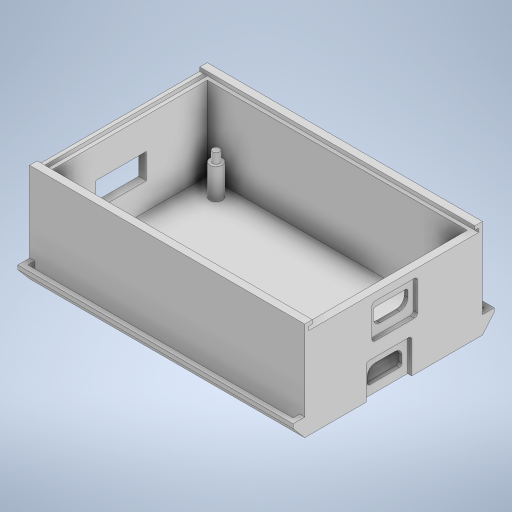
# Autodesk Inventor part: ControllerChassis
Saved by Autodesk Inventor 2024 (Build 280153000, 153)
## iProperties
Created: 2024-03-27
Part Number: ControllerChassis
Material: Generic
Document SubType Name: Modeling
Designer: bbbmi
Density: 1 g/cm^3
Appearance: Default
Author: bbbmi
Autodesk Inventor part; units mm, degrees
ref_plane "YZ Plane" through (0, 0, 0) normal (1, 0, 0) x (0, 1, 0)
ref_plane "XZ Plane" through (0, 0, 0) normal (0, 1, 0) x (-1, 0, 0)
ref_plane "XY Plane" through (0, 0, 0) normal (0, 0, 1) x (1, 0, 0)
sketch "Sketch1" plane through (0, 0, 0) normal (0, 1, 0) x (-1, 0, 0)
  circle A0 centre (57.0611, -2.9464) radius 0.889
  circle A1 centre (57.0611, -36.957) radius 0.889
  circle A2 centre (2.9464, -2.9464) radius 0.889
  circle A3 centre (2.9464, -36.957) radius 0.889
  line L0 (0, -39.9034) -> (-2.0828, -39.9034)
  line L1 (-2.0828, 0) -> (-2.0828, -39.9034)
  line L2 (-2.0828, 0) -> (-2.0828, -39.9034)
  line L3 (-2.0828, -39.9034) -> (62.2173, -39.9034)
  line L4 (62.2173, -39.9034) -> (62.2173, 0)
  line L5 (-2.0828, 0) -> (62.2173, 0)
  line L6 (62.6142, 0.3969) -> (62.6142, -40.3003)
  line L7 (62.6142, -40.3003) -> (-2.4797, -40.3003)
  line L8 (-2.4797, -40.3003) -> (-2.4797, 0.3969)
  line L9 (-2.4797, 0.3969) -> (62.6142, 0.3969)
  circle A4 centre (2.9464, -2.9464) radius 1.5875
  circle A5 centre (2.9464, -36.957) radius 1.5875
  circle A6 centre (57.0611, -36.957) radius 1.5875
  circle A7 centre (57.0611, -2.9464) radius 1.5875
  line L10 (64.5192, -42.2053) -> (64.5192, 2.3019)
  line L11 (64.5192, 2.3019) -> (-4.3847, 2.3019)
  line L12 (-4.3847, 2.3019) -> (-4.3847, -42.2053)
  line L13 (-4.3847, -42.2053) -> (64.5192, -42.2053)
  point P0 (0, 0)
  dimension "d3" = 1.778
  dimension "d4" = 1.778
  dimension "d5" = 1.778
  dimension "d6" = 1.778
  dimension "d7" = 2.0828
  dimension "d9" = 0.3969
  dimension "d10" = 3.175
  dimension "d11" = 3.175
  dimension "d12" = 3.175
  dimension "d13" = 3.175
  dimension "d14" = 65.0939
  dimension "d15" = 1.905
  constraints: 28 end point, 8 centre point, 4 coincident, 3 parallel, 3 perpendicular, 6 other
  measures "d3" diameter of A0
  measures "d4" diameter of A1
  measures "d5" diameter of A2
  measures "d6" diameter of A3
  measures "d7" distance of L0.start L0.end
  measures "d9" distance between parallel lines of L5 L9
  measures "d10" diameter of A4
  measures "d11" diameter of A5
  measures "d12" diameter of A6
  measures "d13" diameter of A7
  measures "d14" distance of L8.end L6.start
  measures "d15" distance between parallel lines of L6 L10
extrude "Extrusion1" add sketch "Sketch1" against normal blind 1.905 contours A0 | A1 | A2 | A3 | L0 L1 L5 L4 L3 | L6 L7 L8 L9 | A4 | A5 | A6 | A7 | L13 L12 L11 L10
extrude "Extrusion2" add sketch "Sketch1" along normal blind 20.32 contours L13 L12 L11 L10
extrude "Extrusion3" add sketch "Sketch1" along normal blind 7.62 contours A0 | A1 | A2 | A3 | A4 | A5 | A6 | A7
extrude "Extrusion4" add sketch "Sketch1" along normal blind 10.16 contours A0 | A1 | A2 | A3
sketch "Sketch2" plane through (-62.6142, 0, -40.3003) normal (1, 0, 0) x (0, 0, -1)
  line L0 (-35.7664, 7.62) -> (-38.9414, 7.62) projected
  line L1 (-1.7558, 7.62) -> (-4.9308, 7.62) projected
  line L2 (-38.9414, 7.62) -> (-1.7558, 7.62) construction
  line L3 (-0.1345, 12.2585) -> (-15.2729, 12.2585) construction
  line L4 (-40.6972, 0) -> (-40.6972, 20.32) construction
  line L5 (-40.6972, 12.2585) -> (-27.9972, 12.2585) construction
  line L6 (-40.6972, 12.2585) -> (-27.9972, 12.2585) construction
  line L7 (-29.9766, 7.62) -> (-29.9766, 12.827) construction
  line L8 (-12.5123, 13.2239) -> (-30.3735, 13.2239) construction
  line L9 (-30.3735, 13.2239) -> (-30.3735, 7.62) construction
  line L10 (-27.9972, 15.5048) -> (-27.9972, 4.9416) construction
  line L11 (-15.2729, 15.5048) -> (-15.2729, 4.9416) construction
  line L12 (-26.1455, 7.62) -> (-26.1455, 6.858) construction
  line L13 (-26.1455, 6.858) -> (-26.1455, 6.4611) construction
  line L14 (-26.1455, 6.4611) -> (-27.9972, 6.4611) construction
  line L15 (-27.9972, 6.4611) -> (-15.2729, 6.4611) construction
  line L16 (-27.9972, 13.2239) -> (-15.2729, 13.2239)
  line L17 (-15.2729, 13.2239) -> (-15.2729, 6.4611)
  line L18 (-15.2729, 6.4611) -> (-27.9972, 6.4611)
  line L19 (-27.9972, 6.4611) -> (-27.9972, 13.2239)
  point P0 (-40.3003, 0)
  dimension "d24" = 15.1384
  dimension "d25" = 12.7
  dimension "d26" = 0
  dimension "d27" = 12.7242
  dimension "d28" = 5.207
  dimension "d30" = 0.762
  dimension "d31" = 0.3969
  constraints: 34 end point, 9 point on line, 6 perpendicular, 3 horizontal, 2 collinear, 2 parallel
  measures "d24" distance of L3.start L3.end
  measures "d25" distance of L5.start L5.end
  measures "d26" distance between parallel lines of L5 L6
  measures "d27" distance of L3.end L5.end
  measures "d28" distance of L7.start L7.end
  measures "d30" distance of L12.start L12.end
  measures "d31" distance of L12.end L13.end
extrude "Extrusion5" cut sketch "Sketch2" against normal blind 10.16
sketch "Sketch3" plane through (-62.6142, 6.4611, -12.3031) normal (0, 1, 0) x (1, 0, 0)
  line L0 (-1.905, 0) -> (-1.905, 12.7242) projected
  line L1 (0, 0) -> (-1.905, 0) projected
  line L2 (0, 12.7242) -> (0, 0) projected
  line L3 (0, 12.7242) -> (-1.905, 12.7242) projected
  point P0 (62.6142, -12.3031)
extrude "Extrusion6" add sketch "Sketch3" along normal blind 0.2032
sketch "Sketch4" plane through (-62.6142, 13.2239, -25.0273) normal (0, -1, 0) x (1, 0, 0)
  line L0 (-1.905, 0) -> (-1.905, 12.7242) projected
  line L1 (0, 0) -> (-1.905, 0) projected
  line L2 (0, 12.7242) -> (0, 0) projected
  line L3 (0, 12.7242) -> (-1.905, 12.7242) projected
  point P0 (62.6142, 25.0273)
extrude "Extrusion7" add sketch "Sketch4" along normal blind 0.2032
sketch "Sketch5" plane through (2.4797, 0, 0.3969) normal (-1, 0, 0) x (0, 0, 1)
  line L0 (-35.7664, 7.62) -> (-38.9414, 7.62) projected
  line L1 (-1.7558, 7.62) -> (-4.9308, 7.62) projected
  line L2 (0, 0) -> (0, 20.32) projected
  line L3 (0, 0) -> (-40.6972, 0) projected
  line L4 (0, 0) -> (0, 20.32) projected
  line L5 (-40.6972, 20.32) -> (0, 20.32) projected
  line L6 (-40.6972, 0) -> (-40.6972, 20.32) projected
  line L7 (0, 17.9413) -> (-16.256, 17.9413) construction
  line L8 (-40.6972, 17.9413) -> (-24.9492, 17.9413) construction
  line L9 (-38.9414, 7.62) -> (-1.7558, 7.62) construction
  line L10 (-31.4008, 7.62) -> (-31.4008, 16.637) construction
  line L11 (-31.4008, 16.637) -> (-9.7411, 16.637) construction
  line L12 (-11.2605, 7.62) -> (-11.2605, 12.5984) construction
  line L13 (-11.2605, 12.5984) -> (-27.4568, 12.5984) construction
  line L14 (-24.9492, 16.002) -> (-24.9492, 11.6374) construction
  line L15 (-16.256, 17.9413) -> (-16.256, 10.1092) construction
  line L16 (-24.3142, 16.637) -> (-16.891, 16.637)
  line L17 (-16.256, 16.002) -> (-16.256, 12.5984)
  line L18 (-16.256, 12.5984) -> (-24.9492, 12.5984)
  line L19 (-24.9492, 12.5984) -> (-24.9492, 16.637)
  arc A0 (-24.9492, 14.6177) -> (-22.9299, 12.5984) centre (-22.9299, 14.6177) ccw
  line L20 (-24.9492, 14.6177) -> (-22.9299, 12.5984) construction
  line L21 (-24.9492, 14.6177) -> (-22.0934, 14.6177) construction
  arc A1 (-17.9578, 12.5984) -> (-16.256, 14.3002) centre (-17.9578, 14.3002) ccw
  line L22 (-16.256, 14.3002) -> (-17.9578, 12.5984) construction
  line L23 (-16.256, 14.3002) -> (-13.8493, 14.3002) construction
  arc A2 (-24.3142, 16.637) -> (-24.9492, 16.002) centre (-24.3142, 16.002) ccw
  arc A3 (-16.256, 16.002) -> (-16.891, 16.637) centre (-16.891, 16.002) ccw
  line L24 (-15.367, 0.4545) -> (-22.7902, 0.4545)
  line L25 (-23.4252, 1.0895) -> (-23.4252, 4.4931)
  line L26 (-23.4252, 4.4931) -> (-14.732, 4.4931)
  line L27 (-14.732, 4.4931) -> (-14.732, 0.4545)
  arc A4 (-14.732, 2.4738) -> (-16.7513, 4.4931) centre (-16.7513, 2.4738) ccw
  line L28 (-14.732, 2.4738) -> (-16.7513, 4.4931) construction
  line L29 (-14.732, 2.4738) -> (-17.5877, 2.4738) construction
  arc A5 (-21.7234, 4.4931) -> (-23.4252, 2.7913) centre (-21.7234, 2.7913) ccw
  line L30 (-23.4252, 2.7913) -> (-21.7234, 4.4931) construction
  arc A6 (-15.367, 0.4545) -> (-14.732, 1.0895) centre (-15.367, 1.0895) ccw
  arc A7 (-23.4252, 1.0895) -> (-22.7902, 0.4545) centre (-22.7902, 1.0895) ccw
  line L31 (-35.7664, 7.62) -> (-35.7664, 3.9878) construction
  line L32 (-40.6972, 3.9878) -> (-23.222, 3.9878) construction
  line L33 (0, 1.7909) -> (-16.3322, 1.7909) construction
  line L34 (-28.4303, 7.62) -> (-28.4303, 0.8509) construction
  line L35 (-28.4303, 0.8509) -> (-22.4064, 0.8509) construction
  line L36 (0, 4.4931) -> (-14.732, 4.4931)
  point P0 (-0.3969, 0)
  point P1 (-14.732, 1.0895)
  dimension "d38" = 16.256
  dimension "d39" = 15.748
  dimension "d40" = 9.017
  dimension "d41" = 4.9784
  dimension "d42" = 45
  dimension "d43" = 135
  dimension "d44" = 0.635
  dimension "d45" = 45
  dimension "d46" = 0.635
  dimension "d47" = 3.6322
  dimension "d48" = 17.4752
  dimension "d49" = 16.3322
  dimension "d50" = 6.7691
  dimension "d157" = 14.732
  constraints: 60 end point, 19 point on line, 16 point on circle, 11 tangent, 10 perpendicular, 8 centre point, 5 horizontal, 4 midpoint, 4 parallel, 4 vertical, 3 equal length, 2 equal radius, 1 collinear
  measures "d38" distance of L7.start L7.end
  measures "d39" distance of L8.start L8.end
  measures "d40" distance of L10.start L10.end
  measures "d41" distance of L12.start L12.end
  measures "d42" angle of L20 L21
  measures "d43" angle of L22 L23
  measures "d44" radius of A2
  measures "d45" angle of L28 L29
  measures "d46" radius of A6
  measures "d47" distance of L0.start L31.end
  measures "d48" distance of L32.start L32.end
  measures "d49" distance of L33.start L33.end
  measures "d50" distance of L34.start L34.end
  measures "d157" distance of L36.start L36.end
extrude "Extrusion8" cut sketch "Sketch5" against normal blind 25.4 contours L16 A3 L17 A1 L18 A0 L19 A2 | L24 A7 L25 A5 L26 A4 L27 A6
sketch "Sketch6" plane through (0, 20.32, 0) normal (0, 1, 0) x (1, 0, 0)
  line L0 (-64.5192, -2.3019) -> (4.3847, -2.3019) projected
  line L1 (4.3847, -2.3019) -> (4.3847, 42.2053) projected
  line L2 (4.3847, 42.2053) -> (-64.5192, 42.2053) projected
  line L3 (-64.5192, 42.2053) -> (-64.5192, -2.3019) projected
  line L4 (-62.6142, -0.3969) -> (-62.6142, 40.3003) projected
  line L5 (-62.6142, 40.3003) -> (2.4797, 40.3003) projected
  line L6 (2.4797, 40.3003) -> (2.4797, -0.3969) projected
  line L7 (2.4797, -0.3969) -> (-62.6142, -0.3969) projected
  point P0 (0, 0)
extrude "Extrusion9" add sketch "Sketch6" along normal blind 0.508
sketch "Sketch7" plane through (0, 20.828, 0) normal (0, 1, 0) x (1, 0, 0)
  line L0 (4.3847, -2.3019) -> (4.3847, 42.2053) projected
  line L1 (4.3847, 42.2053) -> (-64.5192, 42.2053) projected
  line L2 (-64.5192, 42.2053) -> (-64.5192, -2.3019) projected
  line L3 (-64.5192, -2.3019) -> (4.3847, -2.3019) projected
  line L4 (-62.6142, -0.3969) -> (-62.6142, 40.3003) projected
  line L5 (-62.6142, 40.3003) -> (2.4797, 40.3003) projected
  line L6 (2.4797, 40.3003) -> (2.4797, -0.3969) projected
  line L7 (2.4797, -0.3969) -> (-62.6142, -0.3969) projected
  line L8 (-63.5667, -1.3494) -> (-63.5667, 41.2528)
  line L9 (-63.5667, 41.2528) -> (3.4322, 41.2528)
  line L10 (3.4322, 41.2528) -> (3.4322, -1.3494)
  line L11 (3.4322, -1.3494) -> (-63.5667, -1.3494)
  line L12 (3.4322, -1.3494) -> (4.3847, -1.3494)
  line L13 (3.4322, 41.2528) -> (4.3847, 41.2528)
  point P0 (0, 0)
  dimension "d55" = 0.9525
  constraints: 12 end point, 3 point on line, 1 perpendicular, 3 other
  measures "d55" distance between parallel lines of L7 L11
extrude "Extrusion10" add sketch "Sketch7" along normal blind 0.9525 contours L3 L2 L1 L0 L13 L9 L8 L11 L12
sketch "Sketch8" plane through (0, 21.7805, 0) normal (0, 1, 0) x (1, 0, 0)
  line L0 (4.3847, -1.3494) -> (-63.5667, -1.3494) projected
  line L1 (2.4688, -1.3494) -> (0.6908, -1.3494)
  arc A0 (0.6908, -1.3494) -> (2.4688, -1.3494) centre (1.5798, -1.3494) ccw
  line L2 (4.3847, 41.2528) -> (-63.5667, 41.2528) projected
  line L3 (2.4688, 41.2528) -> (0.6908, 41.2528)
  arc A1 (2.4688, 41.2528) -> (0.6908, 41.2528) centre (1.5798, 41.2528) ccw
  point P0 (0, 0)
  dimension "d58" = 1.778
  dimension "d59" = 0.889
  dimension "d60" = 1.778
  dimension "d61" = 0.889
  constraints: 4 end point, 4 point on circle, 4 point on line, 2 centre point
  measures "d58" distance of L1.start L1.end
  measures "d59" radius of A0
  measures "d60" distance of L3.start L3.end
  measures "d61" radius of A1
extrude "Extrusion11" cut sketch "Sketch8" against normal blind 0.9525
sketch "Sketch9" plane through (0, 21.7805, 0) normal (0, 1, 0) x (1, 0, 0)
  line L0 (-62.6142, -0.3969) -> (-62.6142, 40.3003) projected
  line L1 (-62.6142, 40.3003) -> (2.4797, 40.3003) projected
  line L2 (2.4797, 40.3003) -> (2.4797, -0.3969) projected
  line L3 (2.4797, -0.3969) -> (-62.6142, -0.3969) projected
  line L4 (4.3847, 41.2528) -> (2.4688, 41.2528) projected
  arc A0 (2.4688, 41.2528) -> (0.6908, 41.2528) centre (1.5798, 41.2528) ccw projected
  line L5 (0.6908, 41.2528) -> (-63.5667, 41.2528) projected
  line L6 (-63.5667, 41.2528) -> (-63.5667, -1.3494) projected
  line L7 (-63.5667, -1.3494) -> (0.6908, -1.3494) projected
  arc A1 (0.6908, -1.3494) -> (2.4688, -1.3494) centre (1.5798, -1.3494) ccw projected
  line L8 (2.4688, -1.3494) -> (4.3847, -1.3494) projected
  line L9 (4.3847, -1.3494) -> (4.3847, 41.2528) projected
  arc A2 (0.6908, -1.3494) -> (2.4688, -1.3494) centre (1.5798, -1.3494) ccw projected
  line L10 (0.6908, -1.3494) -> (-63.5667, -1.3494) projected
  line L11 (-63.5667, -1.3494) -> (-63.5667, 41.2528) projected
  line L12 (-63.5667, 41.2528) -> (0.6908, 41.2528) projected
  arc A3 (2.4688, 41.2528) -> (0.6908, 41.2528) centre (1.5798, 41.2528) ccw projected
  line L13 (2.4688, 41.2528) -> (4.3847, 41.2528) projected
  line L14 (4.3847, 41.2528) -> (4.3847, 42.2053) projected
  line L15 (4.3847, 42.2053) -> (-64.5192, 42.2053) projected
  line L16 (-64.5192, 42.2053) -> (-64.5192, -2.3019) projected
  line L17 (-64.5192, -2.3019) -> (4.3847, -2.3019) projected
  line L18 (4.3847, -2.3019) -> (4.3847, -1.3494) projected
  line L19 (4.3847, -1.3494) -> (2.4688, -1.3494) projected
  line L20 (2.4797, -0.3969) -> (4.3847, -0.3969)
  line L21 (2.4797, 40.3003) -> (-62.6142, 40.3003) projected
  line L22 (2.4797, 40.3003) -> (4.3847, 40.3003)
  line L23 (-63.5667, 41.2528) -> (-64.5192, 41.2528)
  line L24 (-64.5192, 42.2053) -> (-64.5192, -2.3019) projected
  line L25 (0.6908, -1.3494) -> (-63.5667, -1.3494) projected
  line L26 (-63.5667, -1.3494) -> (-64.5497, -1.3494)
  line L27 (-62.6142, 40.3003) -> (-64.5192, 40.3003)
  line L28 (-62.6142, 40.3003) -> (-60.7092, 40.3003) construction
  line L29 (-62.6142, -0.3969) -> (-62.6142, 40.3003) projected
  line L30 (-62.6142, -0.3969) -> (-64.5192, -0.3969)
  line L31 (-62.6142, -0.3969) -> (-60.7092, -0.3969) construction
  point P0 (0, 0)
  dimension "d64" = 180
  dimension "d65" = 180
  constraints: 16 end point, 5 point on line, 3 perpendicular, 2 collinear, 2 horizontal, 1 parallel
  measures "d64" angle of L27 L28
  measures "d65" angle of L30 L31
extrude "Extrusion12" add sketch "Sketch9" along normal blind 0.9525 contours L3 L20 L9 L8 A1 L7 L6 L30 | L27 L6 L5 A0 L4 L9 L22 L1 | L6 L26 L16 L30 | L27 L16 L23 L6 | L7 A1 L8 L18 L17 L16 L26 | L23 L16 L15 L14 L4 A0 L5
sketch "Sketch10" plane through (4.3847, -1.905, 2.3019) normal (1, 0, 0) x (0, 0, -1)
  line L0 (0, 0) -> (0, 24.638) projected
  line L1 (0, 0) -> (0, 4.4819)
  line L2 (-2.921, 4.4819) -> (-2.921, 3.4361)
  line L3 (-2.921, 3.4361) -> (0, 0)
  line L4 (-2.921, 4.4819) -> (-1.651, 4.4819)
  line L5 (-1.1001, 3.255) -> (0, 1.9608)
  line L6 (-1.1001, 3.255) -> (-1.651, 3.903)
  line L7 (-1.651, 3.903) -> (-1.651, 4.4819)
  line L8 (-1.651, 3.903) -> (0, 1.9608)
  line L9 (-1.651, 4.4819) -> (-2.921, 4.4819)
  line L10 (44.5071, 0) -> (44.5071, 4.4819)
  line L11 (47.4281, 4.4819) -> (47.4281, 3.4361)
  line L12 (47.4281, 3.4361) -> (44.5071, 0)
  line L13 (47.4281, 4.4819) -> (46.1581, 4.4819)
  line L14 (45.6073, 3.255) -> (44.5071, 1.9608)
  line L15 (45.6073, 3.255) -> (46.1581, 3.903)
  line L16 (46.1581, 3.903) -> (46.1581, 4.4819)
  line L17 (46.1581, 3.903) -> (44.5071, 1.9608)
  line L18 (46.1581, 4.4819) -> (47.4281, 4.4819)
  point P0 (2.3019, 1.905)
  point P1 (0, 1.9608)
  dimension "d69" = 2.921
  dimension "d70" = 1.27
  constraints: 36 end point, 5 point on line, 2 perpendicular, 1 collinear
  measures "d69" distance of L1.end L2.start
  measures "d70" distance of L2.start L4.end
extrude "Extrusion13" add sketch "Sketch10" against normal up to surface (68.9039 mm away)
sketch "Sketch11" plane through (4.3847, 20.828, 1.3494) normal (1, 0, 0) x (0, 0, -1)
  line L0 (-2.6035, -18.83) -> (-2.6035, -18.2511) projected
  line L1 (-0.9525, -20.7722) -> (-2.6035, -18.83) projected
  line L2 (-0.9525, -20.7722) -> (-0.9525, 1.905) projected
  line L3 (45.2056, -18.2511) -> (45.2056, -18.83) projected
  line L4 (45.2056, -18.83) -> (43.5546, -20.7722) projected
  line L5 (43.5546, -20.7722) -> (43.5546, 1.905) projected
  line L6 (45.2056, -18.2511) -> (43.5546, -18.2511)
  line L7 (-2.6035, -18.2511) -> (-3.8735, -18.2511) projected
  line L8 (-2.6035, -18.2511) -> (-0.9525, -18.2511)
  point P0 (1.3494, -20.828)
  constraints: 4 end point, 2 perpendicular, 2 point on line
extrude "Extrusion14" add sketch "Sketch11" against normal blind 1.27
sketch "Sketch12" plane through (-64.5192, 21.7805, -40.3003) normal (-1, 0, 0) x (0, 0, 1)
  line L0 (44.2531, -19.7825) -> (42.6021, -21.7247) projected
  line L1 (44.2531, -19.2036) -> (44.2531, -19.7825) projected
  line L2 (44.2531, -19.2036) -> (42.6021, -19.2036) projected
  line L3 (42.6021, -21.7247) -> (42.6021, -19.2036) projected
  line L4 (-3.556, -19.7825) -> (-3.556, -19.2036) projected
  line L5 (-1.905, -21.7247) -> (-3.556, -19.7825) projected
  line L6 (-1.905, -19.2036) -> (-1.905, -21.7247) projected
  line L7 (-1.905, -19.2036) -> (-3.556, -19.2036) projected
  point P0 (40.3003, -21.7805)
extrude "Extrusion15" add sketch "Sketch12" against normal blind 1.27
sketch "Sketch13" plane through (0, -1.905, 0) normal (0, -1, 0) x (1, 0, 0)
  line L0 (4.3847, 2.3019) -> (-64.5192, 2.3019) projected
  line L1 (-64.5192, 2.3019) -> (-64.5192, -42.2053) projected
  line L2 (-64.5192, -42.2053) -> (4.3847, -42.2053) projected
  line L3 (4.3847, -42.2053) -> (4.3847, 2.3019) projected
  circle A0 centre (-30.0673, -19.9517) radius 3.81
  circle A1 centre (-17.3673, -19.9517) radius 3.81
  circle A2 centre (-4.6673, -19.9517) radius 3.81
  circle A3 centre (-30.0673, -32.6517) radius 3.81
  circle A4 centre (-17.3673, -32.6517) radius 3.81
  circle A5 centre (-4.6673, -32.6517) radius 3.81
  circle A6 centre (-17.3673, -32.6517) radius 3.81
  circle A7 centre (-30.0673, -32.6517) radius 3.81
  circle A8 centre (-42.7673, -32.6517) radius 3.81
  circle A9 centre (-55.4673, -32.6517) radius 3.81
  circle A10 centre (-4.6673, -19.9517) radius 3.81
  circle A11 centre (-17.3673, -19.9517) radius 3.81
  circle A12 centre (-30.0673, -19.9517) radius 3.81
  circle A13 centre (-42.7673, -19.9517) radius 3.81
  circle A14 centre (-55.4673, -19.9517) radius 3.81
  circle A15 centre (-4.6673, -7.2517) radius 3.81
  circle A16 centre (-17.3673, -7.2517) radius 3.81
  circle A17 centre (-30.0673, -7.2517) radius 3.81
  circle A18 centre (-42.7673, -7.2517) radius 3.81
  circle A19 centre (-55.4673, -7.2517) radius 3.81
  point P0 (0, 0)
  dimension "d83" = 12.7
  dimension "d86" = 12.7
  dimension "d91" = 12.7
  dimension "d94" = 12.7
  constraints: 20 centre point, 2 horizontal, 2 vertical, 38 other
  measures "d83" distance of A0.centre A1.centre
  measures "d86" distance of A0.centre A3.centre
  measures "d91" distance of A5.centre A6.centre
  measures "d94" distance of A5.centre A10.centre
extrude "Extrusion16" add sketch "Sketch13" along normal blind 2.54 contours A0 | A1 | A2 | A3 | A4 | A5 | A8 | A9 | A13 | A14 | A15 | A16 | A17 | A18 | A19
chamfer "Chamfer1" distance 3.556 distance2 2.54 1 edges at (-8.4773, -4.445, -19.9517) measured on face at (-7.9773, -4.445, -19.9517)
chamfer "Chamfer2" distance 3.556 distance2 2.54 1 edges at (-8.4773, -4.445, -32.6517) measured on face at (-7.9773, -4.445, -32.6517)
chamfer "Chamfer3" distance 3.556 distance2 2.54 1 edges at (-21.1773, -4.445, -32.6517) measured on face at (-20.6773, -4.445, -32.6517)
chamfer "Chamfer4" distance 3.556 distance2 2.54 1 edges at (-33.8773, -4.445, -32.6517) measured on face at (-33.3773, -4.445, -32.6517)
chamfer "Chamfer5" distance 3.556 distance2 2.54 1 edges at (-46.5773, -4.445, -32.6517) measured on face at (-46.0773, -4.445, -32.6517)
chamfer "Chamfer6" distance 3.556 distance2 2.54 1 edges at (-59.2773, -4.445, -32.6517) measured on face at (-58.7773, -4.445, -32.6517)
chamfer "Chamfer7" distance 3.556 distance2 2.54 1 edges at (-21.1773, -4.445, -19.9517) measured on face at (-20.6773, -4.445, -19.9517)
chamfer "Chamfer8" distance 3.556 distance2 2.54 1 edges at (-33.8773, -4.445, -19.9517) measured on face at (-33.3773, -4.445, -19.9517)
chamfer "Chamfer9" distance 3.556 distance2 2.54 1 edges at (-46.5773, -4.445, -19.9517) measured on face at (-46.0773, -4.445, -19.9517)
chamfer "Chamfer10" distance 3.556 distance2 2.54 1 edges at (-8.4773, -4.445, -7.2517) measured on face at (-7.9773, -4.445, -7.2517)
chamfer "Chamfer11" distance 3.556 distance2 2.54 1 edges at (-21.1773, -4.445, -7.2517) measured on face at (-20.6773, -4.445, -7.2517)
chamfer "Chamfer12" distance 3.556 distance2 2.54 1 edges at (-33.8773, -4.445, -7.2517) measured on face at (-33.3773, -4.445, -7.2517)
chamfer "Chamfer13" distance 3.556 distance2 2.54 1 edges at (-59.2773, -4.445, -19.9517) measured on face at (-58.7773, -4.445, -19.9517)
chamfer "Chamfer14" distance 3.556 distance2 2.54 1 edges at (-46.5773, -4.445, -7.2517) measured on face at (-46.0773, -4.445, -7.2517)
chamfer "Chamfer15" distance 3.556 distance2 2.54 1 edges at (-59.2773, -4.445, -7.2517) measured on face at (-58.7773, -4.445, -7.2517)
sketch "Sketch14" plane through (0, -1.905, 0) normal (0, -1, 0) x (1, 0, 0)
  circle A0 centre (-55.4673, -32.6517) radius 3.81 projected
  circle A1 centre (-30.0673, -7.2517) radius 3.81 projected
  circle A2 centre (-17.3673, -19.9517) radius 3.81 projected
  circle A3 centre (-4.6673, -32.6517) radius 3.81 projected
  circle A4 centre (-17.3673, -7.2517) radius 3.81 projected
  circle A5 centre (-30.0673, -19.9517) radius 3.81 projected
  circle A6 centre (-42.7673, -32.6517) radius 3.81 projected
  circle A7 centre (-55.4673, -19.9517) radius 3.81 projected
  circle A8 centre (-42.7673, -7.2517) radius 3.81 projected
  circle A9 centre (-17.3673, -32.6517) radius 3.81 projected
  circle A10 centre (-4.6673, -19.9517) radius 3.81 projected
  circle A11 centre (-4.6673, -7.2517) radius 3.81 projected
  circle A12 centre (-30.0673, -32.6517) radius 3.81 projected
  circle A13 centre (-42.7673, -19.9517) radius 3.81 projected
  circle A14 centre (-55.4673, -7.2517) radius 3.81 projected
  line L0 (4.3847, 2.3019) -> (-64.5192, 2.3019) projected
  line L1 (-64.5192, 2.3019) -> (-64.5192, -42.2053) projected
  line L2 (-64.5192, -42.2053) -> (4.3847, -42.2053) projected
  line L3 (4.3847, -42.2053) -> (4.3847, 2.3019) projected
  point P0 (0, 0)
sketch "Sketch15" plane through (4.3847, 20.828, 1.3494) normal (1, 0, 0) x (0, 0, -1)
  line L0 (15.6845, -19.7385) -> (15.6845, -18.3542) projected
  arc A0 (17.7038, -16.3349) -> (15.6845, -18.3542) centre (17.7038, -18.3542) ccw projected
  line L1 (17.7038, -16.3349) -> (22.6759, -16.3349) projected
  arc A1 (24.3777, -18.0367) -> (22.6759, -16.3349) centre (22.6759, -18.0367) ccw projected
  line L2 (24.3777, -18.0367) -> (24.3777, -19.7385) projected
  arc A2 (23.7427, -20.3735) -> (24.3777, -19.7385) centre (23.7427, -19.7385) ccw projected
  line L3 (23.7427, -20.3735) -> (16.3195, -20.3735) projected
  arc A3 (15.6845, -19.7385) -> (16.3195, -20.3735) centre (16.3195, -19.7385) ccw projected
  line L4 (25.9017, -4.826) -> (25.9017, -6.2103) projected
  arc A4 (23.8824, -8.2296) -> (25.9017, -6.2103) centre (23.8824, -6.2103) ccw projected
  line L5 (23.8824, -8.2296) -> (18.9103, -8.2296) projected
  arc A5 (17.2085, -6.5278) -> (18.9103, -8.2296) centre (18.9103, -6.5278) ccw projected
  line L6 (17.2085, -6.5278) -> (17.2085, -4.826) projected
  arc A6 (17.8435, -4.191) -> (17.2085, -4.826) centre (17.8435, -4.826) ccw projected
  line L7 (17.8435, -4.191) -> (25.2667, -4.191) projected
  arc A7 (25.9017, -4.826) -> (25.2667, -4.191) centre (25.2667, -4.826) ccw projected
  line L8 (43.5546, -22.733) -> (-0.9525, -22.733) projected
  line L9 (43.5546, -22.733) -> (46.4756, -19.2969) projected
  line L10 (46.4756, -19.2969) -> (46.4756, -18.2511) projected
  line L11 (46.4756, -18.2511) -> (43.5546, -18.2511) projected
  line L12 (43.5546, -18.2511) -> (43.5546, 1.905) projected
  line L13 (41.6497, 1.905) -> (43.5546, 1.905) projected
  line L14 (41.6497, 0.9525) -> (41.6497, 1.905) projected
  line L15 (41.6497, 0.9525) -> (42.6022, 0.9525) projected
  line L16 (42.6022, 0) -> (42.6022, 0.9525) projected
  line L17 (0, 0) -> (42.6022, 0) projected
  line L18 (0, 0) -> (0, 0.9525) projected
  line L19 (0, 0.9525) -> (0.9525, 0.9525) projected
  line L20 (0.9525, 0.9525) -> (0.9525, 1.905) projected
  line L21 (-0.9525, 1.905) -> (0.9525, 1.905) projected
  line L22 (-0.9525, -18.2511) -> (-0.9525, 1.905) projected
  line L23 (-0.9525, -18.2511) -> (-3.8735, -18.2511) projected
  line L24 (-3.8735, -18.2511) -> (-3.8735, -19.2969) projected
  line L25 (-3.8735, -19.2969) -> (-0.9525, -22.733) projected
  point P0 (1.3494, -20.828)
sketch "Sketch16" plane through (0, 20.828, 0) normal (0, 1, 0) x (1, 0, 0)
  line L0 (-62.6142, -0.3969) -> (-62.6142, 40.3003) projected
  line L1 (-62.6142, 40.3003) -> (2.4797, 40.3003) projected
  line L2 (2.4797, 40.3003) -> (2.4797, -0.3969) projected
  line L3 (2.4797, -0.3969) -> (-62.6142, -0.3969) projected
  line L4 (4.3847, 41.2528) -> (2.4688, 41.2528) projected
  arc A0 (2.4688, 41.2528) -> (0.6908, 41.2528) centre (1.5798, 41.2528) ccw projected
  line L5 (0.6908, 41.2528) -> (-63.5667, 41.2528) projected
  line L6 (-63.5667, 41.2528) -> (-63.5667, -1.3494) projected
  line L7 (-63.5667, -1.3494) -> (0.6908, -1.3494) projected
  arc A1 (0.6908, -1.3494) -> (2.4688, -1.3494) centre (1.5798, -1.3494) ccw projected
  line L8 (2.4688, -1.3494) -> (4.3847, -1.3494) projected
  line L9 (4.3847, -1.3494) -> (4.3847, 41.2528) projected
  point P0 (0, 0)
sketch "Sketch17" plane through (4.3847, 20.828, 1.3494) normal (1, 0, 0) x (0, 0, -1)
  line L0 (15.6845, -19.7385) -> (15.6845, -18.3542) projected
  arc A0 (17.7038, -16.3349) -> (15.6845, -18.3542) centre (17.7038, -18.3542) ccw projected
  line L1 (17.7038, -16.3349) -> (22.6759, -16.3349) projected
  arc A1 (24.3777, -18.0367) -> (22.6759, -16.3349) centre (22.6759, -18.0367) ccw projected
  line L2 (24.3777, -18.0367) -> (24.3777, -19.7385) projected
  arc A2 (23.7427, -20.3735) -> (24.3777, -19.7385) centre (23.7427, -19.7385) ccw projected
  line L3 (23.7427, -20.3735) -> (16.3195, -20.3735) projected
  arc A3 (15.6845, -19.7385) -> (16.3195, -20.3735) centre (16.3195, -19.7385) ccw projected
  line L4 (25.9017, -4.826) -> (25.9017, -6.2103) projected
  arc A4 (23.8824, -8.2296) -> (25.9017, -6.2103) centre (23.8824, -6.2103) ccw projected
  line L5 (23.8824, -8.2296) -> (18.9103, -8.2296) projected
  arc A5 (17.2085, -6.5278) -> (18.9103, -8.2296) centre (18.9103, -6.5278) ccw projected
  line L6 (17.2085, -6.5278) -> (17.2085, -4.826) projected
  arc A6 (17.8435, -4.191) -> (17.2085, -4.826) centre (17.8435, -4.826) ccw projected
  line L7 (17.8435, -4.191) -> (25.2667, -4.191) projected
  arc A7 (25.9017, -4.826) -> (25.2667, -4.191) centre (25.2667, -4.826) ccw projected
  line L8 (43.5546, -22.733) -> (-0.9525, -22.733) projected
  line L9 (43.5546, -22.733) -> (46.4756, -19.2969) projected
  line L10 (46.4756, -19.2969) -> (46.4756, -18.2511) projected
  line L11 (46.4756, -18.2511) -> (43.5546, -18.2511) projected
  line L12 (43.5546, -18.2511) -> (43.5546, 1.905) projected
  line L13 (41.6497, 1.905) -> (43.5546, 1.905) projected
  line L14 (41.6497, 0.9525) -> (41.6497, 1.905) projected
  line L15 (41.6497, 0.9525) -> (42.6022, 0.9525) projected
  line L16 (42.6022, 0) -> (42.6022, 0.9525) projected
  line L17 (0, 0) -> (42.6022, 0) projected
  line L18 (0, 0) -> (0, 0.9525) projected
  line L19 (0, 0.9525) -> (0.9525, 0.9525) projected
  line L20 (0.9525, 0.9525) -> (0.9525, 1.905) projected
  line L21 (-0.9525, 1.905) -> (0.9525, 1.905) projected
  line L22 (-0.9525, -18.2511) -> (-0.9525, 1.905) projected
  line L23 (-0.9525, -18.2511) -> (-3.8735, -18.2511) projected
  line L24 (-3.8735, -18.2511) -> (-3.8735, -19.2969) projected
  line L25 (-3.8735, -19.2969) -> (-0.9525, -22.733) projected
  line L26 (20.1898, -16.3349) -> (20.1898, -20.3735)
  line L27 (20.1898, -18.3542) -> (25.9048, -18.3542)
  line L28 (25.0664, -14.0362) -> (15.1604, -14.0362)
  line L29 (14.3984, -14.7982) -> (14.3984, -22.6722)
  line L30 (17.0176, -22.6722) -> (17.0176, -22.733)
  line L31 (43.5546, -22.733) -> (-0.9525, -22.733) projected
  line L32 (28.4446, -22.6722) -> (28.4446, -22.733)
  line L33 (25.8284, -22.733) -> (14.3984, -22.733)
  line L34 (21.5551, -4.191) -> (21.5551, -8.2296)
  line L35 (21.5551, -6.2103) -> (27.2701, -6.2103)
  line L36 (27.2701, -6.2103) -> (27.2701, -1.8923)
  line L37 (26.5081, -1.8923) -> (16.6021, -1.8923)
  line L38 (15.8401, -2.6543) -> (15.8401, -9.7663)
  line L39 (16.6021, -10.5283) -> (26.5081, -10.5283)
  line L40 (27.2701, -9.7663) -> (27.2701, -2.6543)
  arc A8 (27.2701, -2.6543) -> (26.5081, -1.8923) centre (26.5081, -2.6543) ccw
  arc A9 (16.6021, -1.8923) -> (15.8401, -2.6543) centre (16.6021, -2.6543) ccw
  arc A10 (15.8401, -9.7663) -> (16.6021, -10.5283) centre (16.6021, -9.7663) ccw
  arc A11 (26.5081, -10.5283) -> (27.2701, -9.7663) centre (26.5081, -9.7663) ccw
  arc A12 (25.8284, -14.7982) -> (25.0664, -14.0362) centre (25.0664, -14.7982) ccw
  arc A13 (15.1604, -14.0362) -> (14.3984, -14.7982) centre (15.1604, -14.7982) ccw
  line L41 (25.8284, -14.7982) -> (25.8284, -22.733)
  line L42 (14.3984, -22.733) -> (25.8284, -22.733)
  line L43 (-0.9525, -22.733) -> (43.5546, -22.733) projected
  point P0 (1.3494, -20.828)
  point P1 (14.3984, -14.0362)
  point P2 (15.8401, -10.5283)
  point P3 (15.8401, -1.8923)
  point P4 (27.2701, -10.5283)
  point P5 (28.4476, -22.6722)
  dimension "d144" = 5.715
  dimension "d146" = 14.0462
  dimension "d147" = 8.636
  dimension "d148" = 5.715
  dimension "d149" = 4.318
  dimension "d150" = 11.43
  dimension "d151" = 8.636
  dimension "d152" = 0.762
  constraints: 32 end point, 12 point on circle, 12 point on line, 11 tangent, 10 perpendicular, 6 centre point, 5 equal radius, 4 midpoint, 2 collinear, 2 horizontal, 2 parallel
  measures "d144" distance of L27.start L27.end
  measures "d146" distance of L32.start L29.end
  measures "d147" distance of L29.end point (14.398, -14.036)
  measures "d148" distance of L35.start L35.end
  measures "d149" distance of L35.end L36.end
  measures "d150" distance of point (27.27, -10.528) point (15.84, -10.528)
  measures "d151" distance of point (15.84, -10.528) point (15.84, -1.892)
  measures "d152" radius of A8
extrude "Extrusion17" cut sketch "Sketch17" against normal blind 1.016 fills toward (25.7784, -18.7656) open curves L41 A12 L28 A13 L29
extrude "Extrusion18" cut sketch "Sketch17" against normal blind 1.016 contours L40 A11 L39 A10 L38 A9 L37 A8 L36
body "Solid1"
